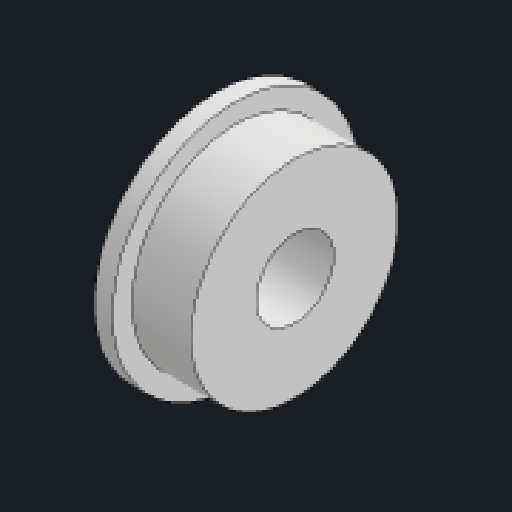
# Autodesk Inventor part: Bearing
Saved by Autodesk Inventor 2023.2 (Build 272271030, 271C)
## iProperties
Created: 2024-02-28
Part Number: Bearing
Material: Generic
Document SubType Name: Modeling
Designer: robpl
Density: 1 g/cm^3
Appearance: Default
Author: robpl
Autodesk Inventor part; units mm, degrees
ref_plane "YZ Plane" through (0, 0, 0) normal (1, 0, 0) x (0, 1, 0)
ref_plane "XZ Plane" through (0, 0, 0) normal (0, 1, 0) x (-1, 0, 0)
ref_plane "XY Plane" through (0, 0, 0) normal (0, 0, 1) x (1, 0, 0)
sketch "Sketch1" plane through (0, 0, 0) normal (0, 0, 1) x (1, 0, 0)
  line L0 (0, 4) -> (3, 4)
  line L1 (3, 4) -> (3, 1.5)
  line L2 (3, 1.5) -> (0, 1.5)
  line L3 (0, 1.5) -> (0, 4)
  line L4 (0, 4) -> (0.7, 4)
  line L5 (0.7, 4) -> (0.7, 4.75)
  line L6 (0.7, 4.75) -> (0, 4.75)
  line L7 (0, 4.75) -> (0, 4)
  line L8 (-0.6, 0) -> (3.6, 0) projected
  point P0 (0, 0)
  dimension "d0" = 3
  dimension "d1" = 4
  dimension "d2" = 1.5
  dimension "d3" = 4.75
  dimension "d4" = 0.7
  constraints: 16 end point, 4 parallel, 2 horizontal, 2 perpendicular, 1 point on line
  measures "d0" distance of L1.end L2.end
  measures "d1" distance from line of point (0, 0) L0
  measures "d2" distance from line of point (0, 0) L2
  measures "d3" distance from line of point (0, 0) L6
  measures "d4" distance of L5.end L6.end
revolve "Revolution1" add sketch "Sketch1" angle 360 about axis through (-10, 0, 0) along (1, 0, 0)
body "Solid1"
